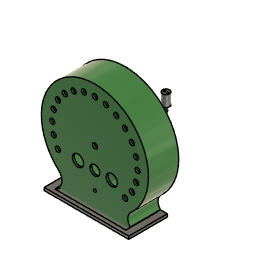
Minutka (Autodesk Fusion 360 design; units mm, degrees)
Autodesk Fusion 360 part; units mm, degrees
note: some values were not read from the file. Set by a fixed rule: which face or edge a step refers to.
sketch "Sketch1" plane through (0, 0, 0) normal (0, 1, 0) x (1, 0, 0)
  circle A0 centre (0, 0) radius 35.5
  circle A1 centre (0, 0) radius 37
  circle A2 centre (0, 0) radius 38
  line L0 (-25, 37.5) -> (25, 37.5)
  line L1 (25, 37.5) -> (25, 39.5)
  line L2 (25, 39.5) -> (-25, 39.5)
  line L3 (-25, 39.5) -> (-25, 37.5)
  arc A3 (-25.5469, 28.131) -> (-25, 37.5) centre (-30.0546, 33.0946) ccw
  arc A4 (25, 37.5) -> (25.5469, 28.131) centre (30.0546, 33.0946) ccw
  dimension "d1" = 71
  dimension "d2" = 74
  dimension "d3" = 76
  dimension "d4" = 50
  dimension "d5" = 2
  dimension "d6" = 37.5
  dimension "d7" = 25
  constraint coincident A0.centre A1.centre
  constraint concentric A1 A2
  constraint horizontal L0
  constraint vertical L1
  constraint horizontal L2
  constraint vertical L3
  constraint tangent A2 A3
  constraint coincident A2 A3.start
  measures "d1" diameter of A0
  measures "d2" diameter of A1
  measures "d3" diameter of A2
  measures "d4" distance of L0.start L0.end
  measures "d5" distance of L0.start L2.end
  measures "d6" vertical distance of A0.centre L0.end
  measures "d7" horizontal distance of A0.centre L0.end
extrude "Extrude1" add sketch "Sketch1" along normal blind 18 contours A2 L0 | A2 L0 A4 | A2 L0 A3 | A2 L0 | A2 L0 L1 L2 L3 makes body 1
extrude "Extrude2" add sketch "Sketch1" along normal blind 17.2 contours A1 bodies 1
extrude "Extrude3" add sketch "Sketch1" along normal blind 0.8 contours A0 bodies 1
sketch "Sketch2" plane through (0, 17.2, 0) normal (0, 1, 0) x (-1, 0, 0)
  circle A0 centre (0, 0) radius 35.5
  circle A1 centre (0, 0) radius 37
  line L0 (-1.5, 38.5) -> (1.5, 38.5)
  line L1 (1.5, 38.5) -> (1.5, 35)
  line L2 (1.5, 35) -> (-1.5, 35)
  line L3 (-1.5, 35) -> (-1.5, 38.5)
  line L4 (-1.5, -42.5) -> (1.5, -42.5)
  line L5 (1.5, -42.5) -> (1.5, -34.5)
  line L6 (1.5, -34.5) -> (-1.5, -34.5)
  line L7 (-1.5, -34.5) -> (-1.5, -42.5)
  constraint horizontal L0
  constraint vertical L1
  constraint horizontal L2
  constraint vertical L3
  constraint horizontal L4
  constraint vertical L5
  constraint horizontal L6
  constraint vertical L7
extrude "Extrude4" cut sketch "Sketch2" against normal blind 1 contours A0 A1 L1 L3 | A0 A1 L5 L7 bodies 1
sketch "Sketch3" plane through (0, 0, 0) normal (0, 1, 0) x (1, 0, 0)
  circle A0 centre (-30.3, 0) radius 1.8
  circle A1 centre (-29.2676, 7.8422) radius 1.8
  circle A2 centre (-26.2406, 15.15) radius 1.8
  circle A3 centre (-29.2676, -7.8422) radius 1.8
  circle A4 centre (-26.2406, -15.15) radius 1.8
  circle A5 centre (-21.4253, -21.4253) radius 1.8
  circle A6 centre (-15.15, -26.2406) radius 1.8
  circle A7 centre (-7.8422, -29.2676) radius 1.8
  circle A8 centre (0, -30.3) radius 1.8
  circle A9 centre (7.8422, -29.2676) radius 1.8
  circle A10 centre (15.15, -26.2406) radius 1.8
  circle A11 centre (21.4253, -21.4253) radius 1.8
  circle A12 centre (26.2406, -15.15) radius 1.8
  circle A13 centre (29.2676, -7.8422) radius 1.8
  circle A14 centre (30.3, 0) radius 1.8
  circle A15 centre (29.2676, 7.8422) radius 1.8
  circle A16 centre (26.2406, 15.15) radius 1.8
  circle A17 centre (21.4253, 21.4253) radius 1.8
  circle A18 centre (0, 0) radius 1.8
  circle A19 centre (0, 27.5) radius 1
  circle A20 centre (0, 15) radius 3.5
  circle A21 centre (-12, 15) radius 4
  circle A22 centre (12, 15) radius 4
  dimension "d16" = 3.6
  dimension "d17" = 30.3
  dimension "d19" = -30
  dimension "d21" = 225
  dimension "d22" = 3.6
  dimension "d23" = 2
  dimension "d24" = 27.5
  dimension "d25" = 7
  dimension "d26" = 15
  dimension "d27" = 8
  dimension "d28" = 12
  dimension "d29" = 8
  dimension "d30" = 12
  constraint coincident A18.centre origin
  measures "d16" diameter of A0
  measures "d17" distance of A18.centre A0.centre
  measures "d22" diameter of A18
  measures "d23" diameter of A19
  measures "d24" distance of A18.centre A19.centre
  measures "d25" diameter of A20
  measures "d26" distance of A18.centre A20.centre
  measures "d27" diameter of A21
  measures "d28" distance of A20.centre A21.centre
  measures "d29" diameter of A22
  measures "d30" distance of A20.centre A22.centre
extrude "Extrude5" cut sketch "Sketch3" along normal blind 0.8 bodies 1
sketch "Sketch4" plane through (0, 0, 0) normal (0, -1, 0) x (1, 0, 0)
  circle A0 centre (12, -15) radius 4
  circle A1 centre (26.2406, -15.15) radius 1.8
  circle A2 centre (26.2406, 15.15) radius 1.8
  circle A3 centre (0, 30.3) radius 1.8
  circle A4 centre (-26.2406, 15.15) radius 1.8
  circle A5 centre (-26.2406, -15.15) radius 1.8
  circle A6 centre (-29.2676, 7.8422) radius 1.8
  circle A7 centre (-7.8422, 29.2676) radius 1.8
  circle A8 centre (21.4253, 21.4253) radius 1.8
  circle A9 centre (29.2676, -7.8422) radius 1.8
  circle A10 centre (0, -15) radius 3.5
  circle A11 centre (-12, -15) radius 4
  circle A12 centre (21.4253, -21.4253) radius 1.8
  circle A13 centre (29.2676, 7.8422) radius 1.8
  circle A14 centre (7.8422, 29.2676) radius 1.8
  circle A15 centre (-21.4253, 21.4253) radius 1.8
  circle A16 centre (-29.2676, -7.8422) radius 1.8
  circle A17 centre (-30.3, 0) radius 1.8
  circle A18 centre (-15.15, 26.2406) radius 1.8
  circle A19 centre (15.15, 26.2406) radius 1.8
  circle A20 centre (30.3, 0) radius 1.8
  circle A21 centre (0, -27.5) radius 1
  circle A22 centre (0, 0) radius 1.8
  line L0 (-25, -39.5) -> (25, -39.5)
  line L1 (25, -39.5) -> (25, -37.5)
  arc A23 (25.5469, -28.131) -> (25, -37.5) centre (30.0546, -33.0946) ccw
  arc A24 (25.5469, -28.131) -> (-25.5469, -28.131) centre (0, 0) ccw
  arc A25 (-25, -37.5) -> (-25.5469, -28.131) centre (-30.0546, -33.0946) ccw
  line L2 (-25, -37.5) -> (-25, -39.5)
  circle A26 centre (-10, -22.5) radius 3
  circle A27 centre (10, -22.5) radius 3
  circle A28 centre (0, 23) radius 3
  circle A29 centre (8, 23) radius 3
  line L3 (35.3713, -6.9908) -> (35.928, -3.0297)
  line L4 (33.3908, -6.7124) -> (35.3713, -6.9908)
  line L5 (33.9475, -2.7513) -> (33.3908, -6.7124)
  line L6 (35.928, -3.0297) -> (33.9475, -2.7513)
  line L7 (-33.9475, 2.7513) -> (-33.3908, 6.7124)
  line L8 (-35.928, 3.0297) -> (-33.9475, 2.7513)
  line L9 (-35.3713, 6.9908) -> (-35.928, 3.0297)
  line L10 (-33.3908, 6.7124) -> (-35.3713, 6.9908)
  dimension "d33" = 6
  dimension "d34" = 22.5
  dimension "d35" = 10
  dimension "d36" = 6
  dimension "d37" = 10
  dimension "d38" = 22.5
  dimension "d39" = 6
  dimension "d40" = 23
  dimension "d41" = 6
  dimension "d42" = 8
  dimension "d115" = 360
  measures "d33" diameter of A26
  measures "d34" vertical distance of A22.centre A26.centre
  measures "d35" horizontal distance of A22.centre A26.centre
  measures "d36" diameter of A27
  measures "d37" horizontal distance of A22.centre A27.centre
  measures "d38" vertical distance of A22.centre A27.centre
  measures "d39" diameter of A28
  measures "d40" distance of A22.centre A28.centre
  measures "d41" diameter of A29
  measures "d42" distance of A28.centre A29.centre
extrude "Extrude6" add sketch "Sketch4" against normal blind 8.8 contours A26 | A29 bodies 1
extrude "Extrude7" add sketch "Sketch4" against normal blind 17.2 contours A27 | A28 bodies 1
sketch "Sketch5" plane through (0, 8.8, 0) normal (0, 1, 0) x (-1, 0, 0)
  circle A0 centre (-8, 23) radius 3
  circle A1 centre (-8, 23) radius 0.9
  circle A2 centre (10, -22.5) radius 0.9
  dimension "d47" = 1.8
  dimension "d48" = 1.8
  constraint concentric A0 A1
  measures "d47" diameter of A1
  measures "d48" diameter of A2
extrude "Extrude8" cut sketch "Sketch5" against normal blind 7 contours A1 | A2 bodies 1
sketch "Sketch6" plane through (0, 17.2, 0) normal (0, 1, 0) x (-1, 0, 0)
  circle A0 centre (0, 23) radius 3
  circle A1 centre (0, 23) radius 1.25
  circle A2 centre (-10, -22.5) radius 1.25
  dimension "d51" = 2.5
  dimension "d52" = 2.5
  constraint concentric A0 A1
  measures "d51" diameter of A1
  measures "d52" diameter of A2
sketch "Sketch7" plane through (0, 0.8, 0) normal (0, 1, 0) x (-1, 0, 0)
  circle A0 centre (-10, -22.5) radius 3
  circle A1 centre (0, 23) radius 3
  circle A2 centre (10, -22.5) radius 3
  circle A3 centre (-8, 23) radius 3
  circle A4 centre (-12, -15) radius 4
  circle A5 centre (-26.2406, -15.15) radius 1.8
  circle A6 centre (-26.2406, 15.15) radius 1.8
  circle A7 centre (0, 30.3) radius 1.8
  circle A8 centre (26.2406, 15.15) radius 1.8
  circle A9 centre (26.2406, -15.15) radius 1.8
  circle A10 centre (29.2676, 7.8422) radius 1.8
  circle A11 centre (7.8422, 29.2676) radius 1.8
  circle A12 centre (-21.4253, 21.4253) radius 1.8
  circle A13 centre (-29.2676, -7.8422) radius 1.8
  circle A14 centre (0, -15) radius 3.5
  circle A15 centre (12, -15) radius 4
  circle A16 centre (-21.4253, -21.4253) radius 1.8
  circle A17 centre (-29.2676, 7.8422) radius 1.8
  circle A18 centre (-7.8422, 29.2676) radius 1.8
  circle A19 centre (21.4253, 21.4253) radius 1.8
  circle A20 centre (29.2676, -7.8422) radius 1.8
  circle A21 centre (30.3, 0) radius 1.8
  circle A22 centre (15.15, 26.2406) radius 1.8
  circle A23 centre (-15.15, 26.2406) radius 1.8
  circle A24 centre (-30.3, 0) radius 1.8
  circle A25 centre (0, -27.5) radius 1
  circle A26 centre (0, 0) radius 1.8
  circle A27 centre (0, 0) radius 35.5
extrude "Extrude9" cut sketch "Sketch6" against normal blind 12 contours A1 | A2 bodies 1
sketch "Sketch8" plane through (0, 17.2, 0) normal (0, 1, 0) x (-1, 0, 0)
  line L0 (-1.5, 35.4683) -> (-1.5, 36.9696)
  arc A0 (-1.5, 36.9696) -> (-1.5, -36.9696) centre (0, 0) ccw
  line L1 (-1.5, -36.9696) -> (-1.5, -35.4683)
  arc A1 (-1.5, 35.4683) -> (-1.5, -35.4683) centre (0, 0) ccw
  circle A2 centre (0, 0) radius 36.5
  line L2 (-1.25, 38.5) -> (1.25, 38.5)
  line L3 (1.25, 38.5) -> (1.25, 34.7673)
  line L4 (1.25, 34.7673) -> (-1.25, 34.7673)
  line L5 (-1.25, 34.7673) -> (-1.25, 38.5)
  circle A3 centre (0, 0) radius 37
  line L6 (-1.25, -34) -> (1.25, -34)
  line L7 (1.25, -34) -> (1.25, -38.157)
  line L8 (1.25, -38.157) -> (-1.25, -38.157)
  line L9 (-1.25, -38.157) -> (-1.25, -34)
  circle A4 centre (-10, -22.5) radius 1.5
  circle A5 centre (0, 23) radius 1.5
  dimension "d55" = 73
  dimension "d56" = 2.5
  dimension "d57" = 1.25
  dimension "d58" = 2.5
  dimension "d59" = 1.25
  dimension "d60" = 3
  dimension "d61" = 3
  constraint coincident A0.centre A1.centre
  constraint horizontal L2
  constraint vertical L3
  constraint horizontal L4
  constraint vertical L5
  constraint horizontal L6
  constraint vertical L7
  constraint horizontal L8
  constraint vertical L9
  measures "d55" diameter of A2
  measures "d56" distance of L2.start L2.end
  measures "d57" horizontal distance of L2.start A0.centre
  measures "d58" distance of L6.start L6.end
  measures "d59" horizontal distance of A0.centre L6.start
  measures "d60" diameter of A4
  measures "d61" diameter of A5
extrude "Extrude10" add sketch "Sketch8" along normal blind 0.8 separate body contours L0 L1 A1 A2 | L0 L1 A1 A2 L3 L4 L5 L6 L7 L9 | A2 L3 L4 L5 | A2 L6 L7 L9 makes body 2
extrude "Extrude11" add sketch "Sketch8" against normal blind 0.5 contours A2 L3 L4 L5 | A2 L6 L7 L9 bodies 2
sketch "Sketch9" plane through (0, 0, 0) normal (0, 0, 1) x (1, 0, 0)
  line L0 (-30, 21, -39.5) -> (30, 21, -39.5)
  line L1 (30, 21, -39.5) -> (30, -6.5, -39.5)
  line L2 (30, -6.5, -39.5) -> (-30, -6.5, -39.5)
  line L3 (-30, -6.5, -39.5) -> (-30, 21, -39.5)
  line L4 (-25.25, 18.25, -39.5) -> (25.25, 18.25, -39.5)
  line L5 (25.25, 18.25, -39.5) -> (25.25, -3.75, -39.5)
  line L6 (25.25, -3.75, -39.5) -> (-25.25, -3.75, -39.5)
  line L7 (-25.25, -3.75, -39.5) -> (-25.25, 18.25, -39.5)
  point P0 (0, 0)
  dimension "d66" = 60
  dimension "d67" = 27.5
  dimension "d70" = 50.5
  dimension "d71" = 22
extrude "Extrude14" add sketch "Sketch9" along normal blind 2 separate body contours L0 L1 L2 L3 in plane through (0, 0, -39.5) normal (0, 0, 1) makes body 3
extrude "Extrude15" add sketch "Sketch9" along normal blind 0.5 contours L4 L5 L6 L7 in plane through (0, 0, -39.5) normal (0, 0, 1) bodies 3
extrude "Extrude16" add 1 faces at (14.1053, 0, -1.2569) along direction (0, -1, 0) blind 0.5 on bodies 1 bodies 1
extrude "Extrude17" add 2 faces at (10.2855, 8.8, 22.8062) (-9.3454, 8.8, -24.6983) along direction (0, 1, 0) blind 1.5 on bodies 1 bodies 1
extrude "Extrude18" add 2 faces at (2.4008, 17.2, 22.7889) (10.6806, 17.2, -24.812) along direction (0, 1, 0) blind 1.5 on bodies 1 bodies 1
extrude "Extrude19" add 1 faces at (18.6639, 18, -34.1351) along direction (0, 1, 0) blind 2 on bodies 1 bodies 1
extrude "Extrude20" add 2 faces at (3.3726, 17.2, -36.2489) (-3.3726, 17.2, -36.2489) along direction (0, 1, 0) blind 1.5 on bodies 1 bodies 1
extrude "Extrude21" add 2 faces at (1.1667, 16.2, -35.9781) (1.1667, 16.2, 35.9781) along direction (0, 1, 0) blind 1.5 on bodies 1 bodies 1
extrude "Extrude22" add 1 faces at (-8.842, 18, -3.5449) along direction (0, 1, 0) blind 0.5 on bodies 2 bodies 2
extrude "Extrude23" add 2 faces at (10.2855, 10.3, 22.8062) (-9.3454, 10.3, -24.6983) along direction (0, 1, 0) blind 1 on bodies 1 bodies 1
extrude "Extrude24" add 2 faces at (10.6806, 18.7, -24.812) (2.4008, 18.7, 22.7889) along direction (0, 1, 0) blind 1 on bodies 1 bodies 1
extrude "Extrude25" add 2 faces at (3.3726, 18.7, -36.2489) (-3.3726, 18.7, -36.2489) along direction (0, 1, 0) blind 1 on bodies 1 bodies 1
extrude "Extrude26" add 1 faces at (1.1667, 17.7, 35.9781) along direction (0, 1, 0) blind 0.5 on bodies 1 bodies 1
extrude "Extrude27" add 1 faces at (1.1667, 17.7, -35.9781) along direction (0, 1, 0) blind 0.5 on bodies 1 bodies 1
extrude "Extrude28" add 1 faces at (18.6639, 20, -34.1351) along direction (0, 1, 0) blind 1 on bodies 1 bodies 1
extrude "Extrude29" add 2 faces at (0.1389, 16.7, 35.3441) (-0.1389, 16.7, -34.8325) along direction (0, -1, 0) blind 0.5 on bodies 2 bodies 2
extrude "Extrude30" add 1 faces at (-8.4167, 3.5833, -39) along direction (0, 0, 1) blind 0.5 on bodies 3 bodies 3
extrude "Extrude31" add sketch "Sketch4" against normal blind 11.3 contours L3 L4 L5 L6 bodies 1
extrude "Extrude32" add sketch "Sketch4" against normal blind 11.3 contours L7 L8 L9 L10 bodies 1
sketch "Sketch10" plane through (0, 0, 0) normal (0, 0, 1) x (1, 0, 0)
  circle A0 centre (-7.5, 35) radius 2.5
  circle A1 centre (-6.2, 35) radius 0.8
  circle A2 centre (-8.8, 35) radius 0.8
  circle A3 centre (-6.4676, 42.8422) radius 2.5
  circle A4 centre (-5.2118, 42.5058) radius 0.8
  circle A5 centre (-7.7233, 43.1787) radius 0.8
  line L0 (-10, 35) -> (-8.947, 43.1621)
  line L1 (-5, 35) -> (-3.9899, 42.5089)
  circle A6 centre (0, 50) radius 2.5
  circle A7 centre (1.3, 50) radius 0.8
  circle A8 centre (-1.3, 50) radius 0.8
  point P0 (22.8, 35)
  dimension "d120" = 5
  dimension "d121" = 30.3
  dimension "d122" = 1.6
  dimension "d123" = 1.3
  dimension "d124" = 1.6
  dimension "d125" = 1.3
  dimension "d127" = -15
  dimension "d130" = 5
  dimension "d131" = 1.6
  dimension "d132" = 1.6
  dimension "d133" = 1.3
  dimension "d134" = 1.3
  constraint coincident A0 L0.start
  constraint coincident A3 L0.end
  constraint tangent A3 L0
  constraint coincident A0 L1.start
  constraint coincident A3 L1.end
  constraint tangent A3 L1
  measures "d120" diameter of A0
  measures "d121" distance of A0.centre P0
  measures "d122" diameter of A1
  measures "d123" distance of A0.centre A1.centre
  measures "d124" diameter of A2
  measures "d125" distance of A0.centre A2.centre
  measures "d130" diameter of A6
  measures "d131" diameter of A7
  measures "d132" diameter of A8
  measures "d133" distance of A6.centre A8.centre
  measures "d134" distance of A6.centre A7.centre
extrude "Extrude33" add sketch "Sketch10" along normal blind 8 separate body contours A0 L0 | A0 A3 L0 L1 | A3 picked at (-7.5133, 36.196) makes body 4
extrude "Extrude34" add sketch "Sketch10" along normal blind 8 separate body contours A6 makes body 5
sketch "Sketch11" plane through (0, 0, 0) normal (0, 0, 1) x (1, 0, 0)
  circle A0 centre (7, 40) radius 3
  circle A1 centre (7, 32) radius 3.5
  dimension "d137" = 6
  dimension "d138" = 7
  measures "d137" diameter of A0
  measures "d138" diameter of A1
extrude "Extrude35" add sketch "Sketch11" along normal blind 5 separate body contours A1 makes body 6
extrude "Extrude36" add sketch "Sketch11" along normal blind 5 separate body contours A0 makes body 7
sketch "Sketch12" plane through (0, 0, 5) normal (0, 0, 1) x (-1, 0, 0)
  circle A0 centre (-7, -40) radius 3
  line L0 (-5.8, -41.7) -> (-8.2, -41.7)
  line L1 (-8.2, -41.7) -> (-8.2, -38.3)
  line L2 (-8.2, -38.3) -> (-5.8, -38.3)
  line L3 (-5.8, -38.3) -> (-5.8, -41.7)
  circle A1 centre (-7, -32) radius 1.75
  point P0 (-7, -40)
  dimension "d143" = 2.4
  dimension "d144" = 3.4
  dimension "d145" = 1.7
  dimension "d146" = 1.2
  dimension "d147" = 3.5
  constraint horizontal L0
  constraint vertical L1
  constraint horizontal L2
  constraint vertical L3
  measures "d143" distance of L0.start L0.end
  measures "d144" distance of L0.start L2.end
  measures "d145" vertical distance of L0.end P0
  measures "d146" horizontal distance of L0.end P0
  measures "d147" diameter of A1
extrude "Extrude37" cut sketch "Sketch12" against normal blind 2.5 contours L0 L1 L2 L3 bodies 7
extrude "Extrude38" cut sketch "Sketch12" against normal blind 2.5 contours A1 bodies 6
chamfer "Chamfer1" distance 0.6 angle 45 2 edges at (4.203, 38.9152, 0) (3.7369, 30.7343, 0) on bodies 6 7
